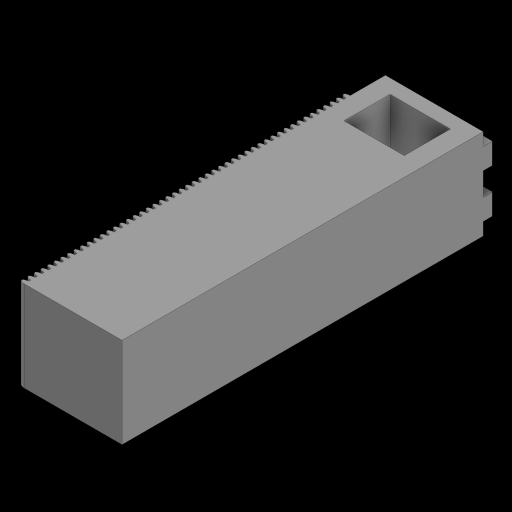
# Autodesk Inventor part: 렉기어
Saved by Autodesk Inventor 2023 (Build 270158000, 158)
## iProperties
Created: 2024-07-04
Part Number: 렉기어
Material: 일반
Document SubType Name: Modeling
Designer: OMS55
Density: 1 g/cm^3
Appearance: 기본값
Mass: 113.431 g
Surface Area: 254.945 cm^2
Volume: 113.431 cm^3
Author: OMS55
Autodesk Inventor part; units mm, degrees
ref_plane "YZ Plane" through (0, 0, 0) normal (1, 0, 0) x (0, 1, 0)
ref_plane "XZ Plane" through (0, 0, 0) normal (0, 1, 0) x (-1, 0, 0)
ref_plane "XY Plane" through (0, 0, 0) normal (0, 0, 1) x (1, 0, 0)
sketch "스케치1" plane through (0, 0, 0) normal (0, 1, 0) x (-1, 0, 0)
  line L0 (0, 0) -> (-34, 0)
  line L1 (-34, 0) -> (-34, -120)
  line L2 (-34, -120) -> (0, -120)
  line L3 (0, -120) -> (0, 0)
  line L4 (-1.5, 0) -> (-34, 0)
  line L5 (-34, 0) -> (-34, -120)
  line L6 (-34, -120) -> (-1.5, -120)
  line L7 (-1.5, -120) -> (-1.5, 0)
  arc A0 (0, -0.477) -> (-1.5, 0) centre (-1.5, -2.597) ccw
  arc A1 (-1.5, -1.454) -> (0, -0.977) centre (-1.5, 1.143) ccw
  line L8 (-1.5, -0.727) -> (0, -0.727) construction
  line L9 (0, -0.477) -> (0, -0.977)
  line L10 (-1.5, 0) -> (-1.5, -1.454)
  arc A2 (0, -2.658) -> (-1.5, -2.181) centre (-1.5, -4.778) ccw
  line L11 (0, -2.658) -> (0, -3.158)
  arc A3 (-1.5, -3.635) -> (0, -3.158) centre (-1.5, -1.038) ccw
  line L12 (-1.5, -2.181) -> (-1.5, -3.635)
  arc A4 (0, -4.839) -> (-1.5, -4.362) centre (-1.5, -6.959) ccw
  line L13 (0, -4.839) -> (0, -5.339)
  arc A5 (-1.5, -5.816) -> (0, -5.339) centre (-1.5, -3.219) ccw
  line L14 (-1.5, -4.362) -> (-1.5, -5.816)
  arc A6 (0, -7.02) -> (-1.5, -6.543) centre (-1.5, -9.14) ccw
  line L15 (0, -7.02) -> (0, -7.52)
  arc A7 (-1.5, -7.997) -> (0, -7.52) centre (-1.5, -5.4) ccw
  line L16 (-1.5, -6.543) -> (-1.5, -7.997)
  arc A8 (0, -9.201) -> (-1.5, -8.724) centre (-1.5, -11.321) ccw
  line L17 (0, -9.201) -> (0, -9.701)
  arc A9 (-1.5, -10.178) -> (0, -9.701) centre (-1.5, -7.581) ccw
  line L18 (-1.5, -8.724) -> (-1.5, -10.178)
  arc A10 (0, -11.382) -> (-1.5, -10.905) centre (-1.5, -13.502) ccw
  line L19 (0, -11.382) -> (0, -11.882)
  arc A11 (-1.5, -12.359) -> (0, -11.882) centre (-1.5, -9.762) ccw
  line L20 (-1.5, -10.905) -> (-1.5, -12.359)
  arc A12 (0, -13.563) -> (-1.5, -13.086) centre (-1.5, -15.683) ccw
  line L21 (0, -13.563) -> (0, -14.063)
  arc A13 (-1.5, -14.54) -> (0, -14.063) centre (-1.5, -11.943) ccw
  line L22 (-1.5, -13.086) -> (-1.5, -14.54)
  arc A14 (0, -15.744) -> (-1.5, -15.267) centre (-1.5, -17.864) ccw
  line L23 (0, -15.744) -> (0, -16.244)
  arc A15 (-1.5, -16.721) -> (0, -16.244) centre (-1.5, -14.124) ccw
  line L24 (-1.5, -15.267) -> (-1.5, -16.721)
  arc A16 (0, -17.925) -> (-1.5, -17.448) centre (-1.5, -20.045) ccw
  line L25 (0, -17.925) -> (0, -18.425)
  arc A17 (-1.5, -18.902) -> (0, -18.425) centre (-1.5, -16.305) ccw
  line L26 (-1.5, -17.448) -> (-1.5, -18.902)
  arc A18 (0, -20.106) -> (-1.5, -19.629) centre (-1.5, -22.226) ccw
  line L27 (0, -20.106) -> (0, -20.606)
  arc A19 (-1.5, -21.083) -> (0, -20.606) centre (-1.5, -18.486) ccw
  line L28 (-1.5, -19.629) -> (-1.5, -21.083)
  arc A20 (0, -22.287) -> (-1.5, -21.81) centre (-1.5, -24.407) ccw
  line L29 (0, -22.287) -> (0, -22.787)
  arc A21 (-1.5, -23.264) -> (0, -22.787) centre (-1.5, -20.667) ccw
  line L30 (-1.5, -21.81) -> (-1.5, -23.264)
  arc A22 (0, -24.468) -> (-1.5, -23.991) centre (-1.5, -26.588) ccw
  line L31 (0, -24.468) -> (0, -24.968)
  arc A23 (-1.5, -25.445) -> (0, -24.968) centre (-1.5, -22.848) ccw
  line L32 (-1.5, -23.991) -> (-1.5, -25.445)
  arc A24 (0, -26.649) -> (-1.5, -26.172) centre (-1.5, -28.769) ccw
  line L33 (0, -26.649) -> (0, -27.149)
  arc A25 (-1.5, -27.626) -> (0, -27.149) centre (-1.5, -25.029) ccw
  line L34 (-1.5, -26.172) -> (-1.5, -27.626)
  arc A26 (0, -28.83) -> (-1.5, -28.353) centre (-1.5, -30.95) ccw
  line L35 (0, -28.83) -> (0, -29.33)
  arc A27 (-1.5, -29.807) -> (0, -29.33) centre (-1.5, -27.21) ccw
  line L36 (-1.5, -28.353) -> (-1.5, -29.807)
  arc A28 (0, -31.011) -> (-1.5, -30.534) centre (-1.5, -33.131) ccw
  line L37 (0, -31.011) -> (0, -31.511)
  arc A29 (-1.5, -31.988) -> (0, -31.511) centre (-1.5, -29.391) ccw
  line L38 (-1.5, -30.534) -> (-1.5, -31.988)
  arc A30 (0, -33.192) -> (-1.5, -32.715) centre (-1.5, -35.312) ccw
  line L39 (0, -33.192) -> (0, -33.692)
  arc A31 (-1.5, -34.169) -> (0, -33.692) centre (-1.5, -31.572) ccw
  line L40 (-1.5, -32.715) -> (-1.5, -34.169)
  arc A32 (0, -35.373) -> (-1.5, -34.896) centre (-1.5, -37.493) ccw
  line L41 (0, -35.373) -> (0, -35.873)
  arc A33 (-1.5, -36.35) -> (0, -35.873) centre (-1.5, -33.753) ccw
  line L42 (-1.5, -34.896) -> (-1.5, -36.35)
  arc A34 (0, -37.554) -> (-1.5, -37.077) centre (-1.5, -39.674) ccw
  line L43 (0, -37.554) -> (0, -38.054)
  arc A35 (-1.5, -38.531) -> (0, -38.054) centre (-1.5, -35.934) ccw
  line L44 (-1.5, -37.077) -> (-1.5, -38.531)
  arc A36 (0, -39.735) -> (-1.5, -39.258) centre (-1.5, -41.855) ccw
  line L45 (0, -39.735) -> (0, -40.235)
  arc A37 (-1.5, -40.712) -> (0, -40.235) centre (-1.5, -38.115) ccw
  line L46 (-1.5, -39.258) -> (-1.5, -40.712)
  arc A38 (0, -41.916) -> (-1.5, -41.439) centre (-1.5, -44.036) ccw
  line L47 (0, -41.916) -> (0, -42.416)
  arc A39 (-1.5, -42.893) -> (0, -42.416) centre (-1.5, -40.296) ccw
  line L48 (-1.5, -41.439) -> (-1.5, -42.893)
  arc A40 (0, -44.097) -> (-1.5, -43.62) centre (-1.5, -46.217) ccw
  line L49 (0, -44.097) -> (0, -44.597)
  arc A41 (-1.5, -45.074) -> (0, -44.597) centre (-1.5, -42.477) ccw
  line L50 (-1.5, -43.62) -> (-1.5, -45.074)
  arc A42 (0, -46.278) -> (-1.5, -45.801) centre (-1.5, -48.398) ccw
  line L51 (0, -46.278) -> (0, -46.778)
  arc A43 (-1.5, -47.255) -> (0, -46.778) centre (-1.5, -44.658) ccw
  line L52 (-1.5, -45.801) -> (-1.5, -47.255)
  arc A44 (0, -48.459) -> (-1.5, -47.982) centre (-1.5, -50.579) ccw
  line L53 (0, -48.459) -> (0, -48.959)
  arc A45 (-1.5, -49.436) -> (0, -48.959) centre (-1.5, -46.839) ccw
  line L54 (-1.5, -47.982) -> (-1.5, -49.436)
  arc A46 (0, -50.64) -> (-1.5, -50.163) centre (-1.5, -52.76) ccw
  line L55 (0, -50.64) -> (0, -51.14)
  arc A47 (-1.5, -51.617) -> (0, -51.14) centre (-1.5, -49.02) ccw
  line L56 (-1.5, -50.163) -> (-1.5, -51.617)
  arc A48 (0, -52.821) -> (-1.5, -52.344) centre (-1.5, -54.941) ccw
  line L57 (0, -52.821) -> (0, -53.321)
  arc A49 (-1.5, -53.798) -> (0, -53.321) centre (-1.5, -51.201) ccw
  line L58 (-1.5, -52.344) -> (-1.5, -53.798)
  arc A50 (0, -55.002) -> (-1.5, -54.525) centre (-1.5, -57.122) ccw
  line L59 (0, -55.002) -> (0, -55.502)
  arc A51 (-1.5, -55.979) -> (0, -55.502) centre (-1.5, -53.382) ccw
  line L60 (-1.5, -54.525) -> (-1.5, -55.979)
  arc A52 (0, -57.183) -> (-1.5, -56.706) centre (-1.5, -59.303) ccw
  line L61 (0, -57.183) -> (0, -57.683)
  arc A53 (-1.5, -58.16) -> (0, -57.683) centre (-1.5, -55.563) ccw
  line L62 (-1.5, -56.706) -> (-1.5, -58.16)
  arc A54 (0, -59.364) -> (-1.5, -58.887) centre (-1.5, -61.484) ccw
  line L63 (0, -59.364) -> (0, -59.864)
  arc A55 (-1.5, -60.341) -> (0, -59.864) centre (-1.5, -57.744) ccw
  line L64 (-1.5, -58.887) -> (-1.5, -60.341)
  arc A56 (0, -61.545) -> (-1.5, -61.068) centre (-1.5, -63.665) ccw
  line L65 (0, -61.545) -> (0, -62.045)
  arc A57 (-1.5, -62.522) -> (0, -62.045) centre (-1.5, -59.925) ccw
  line L66 (-1.5, -61.068) -> (-1.5, -62.522)
  arc A58 (0, -63.726) -> (-1.5, -63.249) centre (-1.5, -65.846) ccw
  line L67 (0, -63.726) -> (0, -64.226)
  arc A59 (-1.5, -64.703) -> (0, -64.226) centre (-1.5, -62.106) ccw
  line L68 (-1.5, -63.249) -> (-1.5, -64.703)
  arc A60 (0, -65.907) -> (-1.5, -65.43) centre (-1.5, -68.027) ccw
  line L69 (0, -65.907) -> (0, -66.407)
  arc A61 (-1.5, -66.884) -> (0, -66.407) centre (-1.5, -64.287) ccw
  line L70 (-1.5, -65.43) -> (-1.5, -66.884)
  arc A62 (0, -68.088) -> (-1.5, -67.611) centre (-1.5, -70.208) ccw
  line L71 (0, -68.088) -> (0, -68.588)
  arc A63 (-1.5, -69.065) -> (0, -68.588) centre (-1.5, -66.468) ccw
  line L72 (-1.5, -67.611) -> (-1.5, -69.065)
  arc A64 (0, -70.269) -> (-1.5, -69.792) centre (-1.5, -72.389) ccw
  line L73 (0, -70.269) -> (0, -70.769)
  arc A65 (-1.5, -71.246) -> (0, -70.769) centre (-1.5, -68.649) ccw
  line L74 (-1.5, -69.792) -> (-1.5, -71.246)
  arc A66 (0, -72.45) -> (-1.5, -71.973) centre (-1.5, -74.57) ccw
  line L75 (0, -72.45) -> (0, -72.95)
  arc A67 (-1.5, -73.427) -> (0, -72.95) centre (-1.5, -70.83) ccw
  line L76 (-1.5, -71.973) -> (-1.5, -73.427)
  arc A68 (0, -74.631) -> (-1.5, -74.154) centre (-1.5, -76.751) ccw
  line L77 (0, -74.631) -> (0, -75.131)
  arc A69 (-1.5, -75.608) -> (0, -75.131) centre (-1.5, -73.011) ccw
  line L78 (-1.5, -74.154) -> (-1.5, -75.608)
  arc A70 (0, -76.812) -> (-1.5, -76.335) centre (-1.5, -78.932) ccw
  line L79 (0, -76.812) -> (0, -77.312)
  arc A71 (-1.5, -77.789) -> (0, -77.312) centre (-1.5, -75.192) ccw
  line L80 (-1.5, -76.335) -> (-1.5, -77.789)
  arc A72 (0, -78.993) -> (-1.5, -78.516) centre (-1.5, -81.113) ccw
  line L81 (0, -78.993) -> (0, -79.493)
  arc A73 (-1.5, -79.97) -> (0, -79.493) centre (-1.5, -77.373) ccw
  line L82 (-1.5, -78.516) -> (-1.5, -79.97)
  arc A74 (0, -81.174) -> (-1.5, -80.697) centre (-1.5, -83.294) ccw
  line L83 (0, -81.174) -> (0, -81.674)
  arc A75 (-1.5, -82.151) -> (0, -81.674) centre (-1.5, -79.554) ccw
  line L84 (-1.5, -80.697) -> (-1.5, -82.151)
  arc A76 (0, -83.355) -> (-1.5, -82.878) centre (-1.5, -85.475) ccw
  line L85 (0, -83.355) -> (0, -83.855)
  arc A77 (-1.5, -84.332) -> (0, -83.855) centre (-1.5, -81.735) ccw
  line L86 (-1.5, -82.878) -> (-1.5, -84.332)
  arc A78 (0, -85.536) -> (-1.5, -85.059) centre (-1.5, -87.656) ccw
  line L87 (0, -85.536) -> (0, -86.036)
  arc A79 (-1.5, -86.513) -> (0, -86.036) centre (-1.5, -83.916) ccw
  line L88 (-1.5, -85.059) -> (-1.5, -86.513)
  arc A80 (0, -87.717) -> (-1.5, -87.24) centre (-1.5, -89.837) ccw
  line L89 (0, -87.717) -> (0, -88.217)
  arc A81 (-1.5, -88.694) -> (0, -88.217) centre (-1.5, -86.097) ccw
  line L90 (-1.5, -87.24) -> (-1.5, -88.694)
  arc A82 (0, -89.898) -> (-1.5, -89.421) centre (-1.5, -92.018) ccw
  line L91 (0, -89.898) -> (0, -90.398)
  arc A83 (-1.5, -90.875) -> (0, -90.398) centre (-1.5, -88.278) ccw
  line L92 (-1.5, -89.421) -> (-1.5, -90.875)
  arc A84 (0, -92.079) -> (-1.5, -91.602) centre (-1.5, -94.199) ccw
  line L93 (0, -92.079) -> (0, -92.579)
  arc A85 (-1.5, -93.056) -> (0, -92.579) centre (-1.5, -90.459) ccw
  line L94 (-1.5, -91.602) -> (-1.5, -93.056)
  arc A86 (0, -94.26) -> (-1.5, -93.783) centre (-1.5, -96.38) ccw
  line L95 (0, -94.26) -> (0, -94.76)
  arc A87 (-1.5, -95.237) -> (0, -94.76) centre (-1.5, -92.64) ccw
  line L96 (-1.5, -93.783) -> (-1.5, -95.237)
  arc A88 (0, -96.441) -> (-1.5, -95.964) centre (-1.5, -98.561) ccw
  line L97 (0, -96.441) -> (0, -96.941)
  arc A89 (-1.5, -97.418) -> (0, -96.941) centre (-1.5, -94.821) ccw
  line L98 (-1.5, -95.964) -> (-1.5, -97.418)
  arc A90 (0, -98.622) -> (-1.5, -98.145) centre (-1.5, -100.742) ccw
  line L99 (0, -98.622) -> (0, -99.122)
  arc A91 (-1.5, -99.599) -> (0, -99.122) centre (-1.5, -97.002) ccw
  line L100 (-1.5, -98.145) -> (-1.5, -99.599)
  arc A92 (0, -100.803) -> (-1.5, -100.326) centre (-1.5, -102.923) ccw
  line L101 (0, -100.803) -> (0, -101.303)
  arc A93 (-1.5, -101.78) -> (0, -101.303) centre (-1.5, -99.183) ccw
  line L102 (-1.5, -100.326) -> (-1.5, -101.78)
  arc A94 (0, -102.984) -> (-1.5, -102.507) centre (-1.5, -105.104) ccw
  line L103 (0, -102.984) -> (0, -103.484)
  arc A95 (-1.5, -103.961) -> (0, -103.484) centre (-1.5, -101.364) ccw
  line L104 (-1.5, -102.507) -> (-1.5, -103.961)
  arc A96 (0, -105.165) -> (-1.5, -104.688) centre (-1.5, -107.285) ccw
  line L105 (0, -105.165) -> (0, -105.665)
  arc A97 (-1.5, -106.142) -> (0, -105.665) centre (-1.5, -103.545) ccw
  line L106 (-1.5, -104.688) -> (-1.5, -106.142)
  arc A98 (0, -107.346) -> (-1.5, -106.869) centre (-1.5, -109.466) ccw
  line L107 (0, -107.346) -> (0, -107.846)
  arc A99 (-1.5, -108.323) -> (0, -107.846) centre (-1.5, -105.726) ccw
  line L108 (-1.5, -106.869) -> (-1.5, -108.323)
  point P0 (-1.5, 0)
  point P1 (-1.5, -120)
  point P2 (-1.5, -84.332)
  point P3 (0, -83.355)
  point P4 (-1.5, -60.341)
  point P5 (0, -59.364)
  point P6 (-1.5, -108.323)
  point P7 (0, -107.346)
  point P8 (-1.5, -106.142)
  point P9 (0, -105.165)
  point P10 (-1.5, -103.961)
  point P11 (0, -102.984)
  point P12 (-1.5, -101.78)
  point P13 (0, -100.803)
  point P14 (-1.5, -99.599)
  point P15 (0, -98.622)
  point P16 (-1.5, -97.418)
  point P17 (0, -96.441)
  point P18 (-1.5, -95.237)
  point P19 (0, -94.26)
  point P20 (-1.5, -93.056)
  point P21 (0, -92.079)
  point P22 (-1.5, -90.875)
  point P23 (0, -89.898)
  point P24 (0, -85.536)
  point P25 (-1.5, -88.694)
  point P26 (-1.5, -82.151)
  point P27 (0, -81.174)
  point P28 (-1.5, -79.97)
  point P29 (0, -78.993)
  point P30 (-1.5, -77.789)
  point P31 (0, -76.812)
  point P32 (-1.5, -75.608)
  point P33 (0, -74.631)
  point P34 (-1.5, -73.427)
  point P35 (0, -72.45)
  point P36 (-1.5, -71.246)
  point P37 (0, -70.269)
  point P38 (-1.5, -69.065)
  point P39 (0, -68.088)
  point P40 (-1.5, -66.884)
  point P41 (0, -65.907)
  point P42 (-1.5, -64.703)
  point P43 (0, -63.726)
  point P44 (-1.5, -62.522)
  point P45 (0, -61.545)
  point P46 (-1.5, -58.16)
  point P47 (0, -57.183)
  point P48 (-1.5, -53.798)
  point P49 (0, -52.821)
  point P50 (-1.5, -51.617)
  point P51 (0, -50.64)
  point P52 (-1.5, -49.436)
  point P53 (0, -48.459)
  point P54 (-1.5, -47.255)
  point P55 (0, -46.278)
  point P56 (-1.5, -45.074)
  point P57 (0, -44.097)
  point P58 (-1.5, -38.531)
  point P59 (0, -37.554)
  point P60 (-1.5, -34.169)
  point P61 (-1.5, -32.715)
  point P62 (-1.5, -29.807)
  point P63 (0, -28.83)
  point P64 (-1.5, -28.353)
  point P65 (-1.5, -25.445)
  point P66 (0, -24.468)
  point P67 (-1.5, -23.991)
  point P68 (-1.5, -23.264)
  point P69 (0, -22.287)
  point P70 (-1.5, -21.81)
  point P71 (-1.5, -55.979)
  point P72 (0, -55.002)
  point P73 (-1.5, -42.893)
  point P74 (0, -41.916)
  point P75 (-1.5, -40.712)
  point P76 (0, -39.735)
  point P77 (-1.5, -36.35)
  point P78 (0, -35.373)
  point P79 (-1.5, -34.896)
  point P80 (-1.5, -31.988)
  point P81 (-1.5, -30.534)
  point P82 (-1.5, -27.626)
  point P83 (0, -26.649)
  point P84 (-1.5, -26.172)
  point P85 (-1.5, -21.083)
  point P86 (0, -20.106)
  point P87 (-1.5, -19.629)
  point P88 (-1.5, -18.902)
  point P89 (-1.5, -16.721)
  point P90 (-1.5, -14.54)
  point P91 (0, -13.563)
  point P92 (-1.5, -13.086)
  point P93 (-1.5, -12.359)
  point P94 (0, -11.382)
  point P95 (-1.5, -10.178)
  point P96 (-1.5, -8.724)
  point P97 (-1.5, -7.997)
  point P98 (0, -7.02)
  point P99 (-1.5, -6.543)
  point P100 (-1.5, -5.816)
  point P101 (0, -4.839)
  point P102 (-1.5, -3.635)
  point P103 (0, -2.658)
  point P104 (-1.5, -2.181)
  point P105 (0, -87.717)
  point P106 (-1.5, -86.513)
  dimension "d0" = 120
  dimension "d1" = 34
  dimension "d2" = 120
  dimension "d3" = 32.5
  dimension "d4" = 1.454
  dimension "d7" = 0.727
  dimension "d8" = 0.25
  dimension "d9" = 0.25
  dimension "d14" = 2.181
  constraints: 294 vertical alignment, 214 end point, 200 point on circle, 100 centre point, 98 collinear, 98 equal radius, 4 vertical, 3 horizontal, 2 parallel, 2 perpendicular, 1 coincident, 1 tangent, 10 other
  measures "d0" distance of L2.end L0.start
  measures "d1" distance of L0.start L0.end
  measures "d2" distance of L6.end L4.start
  measures "d3" distance of L0.end L4.start
  measures "d4" distance of L10.end L4.start
  measures "d7" distance of L8.start L4.start
  measures "d8" distance of L8.end L9.start
  measures "d9" distance of L8.end L9.end
  measures "d14" distance of A0.centre A2.centre
extrude "돌출1" add sketch "스케치1" along normal blind 30 contours L7 L2 L1 L0 | A0 L3 A1 L7 | A2 L3 A3 L7 | L7 A98 L3 A99 | A4 L3 A5 L7 | L7 A96 L3 A97 | A6 L3 A7 L7 | L7 A94 L3 A95 | A8 L3 A9 L7 | L7 A92 L3 A93 | A10 L3 A11 L7 | L7 A90 L3 A91 | A12 L3 A13 L7 | L7 A88 L3 A89 | A14 L3 A15 L7 | L7 A86 L3 A87 | A16 L3 A17 L7 | L7 A84 L3 A85 | A18 L3 A19 L7 | L7 A82 L3 A83 | A20 L3 A21 L7 | L7 A80 L3 A81 | A22 L3 A23 L7 | L7 A79 L3 A80 | L7 A78 L3 A79 | A24 L3 A25 L7 | L7 A76 L3 A77 | A26 L3 A27 L7 | L7 A74 L3 A75 | A28 L3 A29 L7 | L7 A72 L3 A73 | A30 L3 A31 L7 | L7 A70 L3 A71 | A32 L3 A33 L7 | L7 A68 L3 A69 | A34 L3 A35 L7 | L7 A66 L3 A67 | A36 L3 A37 L7 | L7 A64 L3 A65 | A38 L3 A39 L7 | L7 A62 L3 A63 | A40 L3 A41 L7 | L7 A60 L3 A61 | A42 L3 A43 L7 | L7 A58 L3 A59 | A44 L3 A45 L7 | L7 A56 L3 A57 | A46 L3 A47 L7 | L7 A54 L3 A55 | A48 L3 A49 L7 | L7 A52 L3 A53 | A50 L3 A51 L7
extrude "돌출2" cut sketch "스케치1" along normal blind 30 contours L7 A79 L3 A80
sketch "스케치2" plane through (34, 0, -120) normal (0, 0, -1) x (-1, 0, 0)
  line L0 (32.5, 25.8) -> (0, 25.8)
  line L1 (0, 25.8) -> (0, 18.8)
  line L2 (0, 18.8) -> (32.5, 18.8)
  line L3 (32.5, 18.8) -> (32.5, 25.8)
  line L4 (32.5, 11.2) -> (0, 11.2)
  line L5 (0, 11.2) -> (0, 4.2)
  line L6 (0, 4.2) -> (32.5, 4.2)
  line L7 (32.5, 4.2) -> (32.5, 11.2)
  line L8 (32.5, 18.8) -> (32.5, 11.2) construction
  line L9 (0, 18.8) -> (0, 11.2) construction
  line L10 (32.5, 0) -> (32.5, 30) construction
  line L11 (0, 0) -> (0, 30) construction
  point P0 (34, 0)
  point P1 (32.5, 15)
  point P2 (32.5, 15)
  dimension "d21" = 7.6
  dimension "d22" = 7
  dimension "d23" = 7
  constraints: 20 end point, 5 parallel, 2 collinear, 2 horizontal, 2 midpoint, 2 perpendicular, 2 point on line, 1 coincident, 1 vertical
  measures "d21" distance between parallel lines of L4 L2
  measures "d22" distance of L2.end L0.start
  measures "d23" distance of L6.end L4.start
extrude "돌출3" add sketch "스케치2" along normal blind 3
sketch "스케치4" plane through (0, 30, 0) normal (0, 1, 0) x (1, 0, 0)
  line L0 (27.75, 115.3) -> (7.75, 115.3)
  line L1 (7.75, 115.3) -> (7.75, 100)
  line L2 (7.75, 100) -> (27.75, 100)
  line L3 (27.75, 100) -> (27.75, 115.3)
  line L4 (34, 120) -> (1.5, 120) projected
  line L5 (34, 0) -> (34, 120) projected
  point P0 (0, 0)
  dimension "d26" = 20
  dimension "d27" = 20
  dimension "d28" = 6.25
  dimension "d29" = 4.7
  constraints: 8 end point, 2 parallel, 1 horizontal, 1 perpendicular
  measures "d26" distance between parallel lines of L2 L4
  measures "d27" distance between parallel lines of L1 L3
  measures "d28" distance between parallel lines of L5 L3
  measures "d29" distance between parallel lines of L4 L0
extrude "돌출4" cut sketch "스케치4" against normal blind 30
sketch "스케치5" plane through (7.75, 30, -115.3) normal (0, 0, 1) x (1, 0, 0)
  circle A0 centre (7.45, -15) radius 1.45
  line L0 (-6.25, -18.8) -> (-6.25, -11.2) projected
  point P0 (-7.75, -30)
  point P1 (-6.25, -15)
  dimension "d33" = 13.7
  constraints: 1 centre point, 1 horizontal alignment, 1 midpoint
  measures "d33" distance from line of L0 A0.centre
extrude "돌출5" cut sketch "스케치5" against normal blind 30
